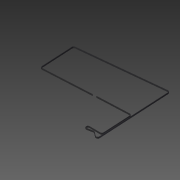
# Autodesk Inventor part: BeltLeft
Saved by Autodesk Inventor 2015 (Build 190159000, 159)
## iProperties
Company: RobotDigg
Created: 2014-08-13
Part Number: BeltLeft
Material: Rubber, Silicone
Document SubType Name: Modeling
Designer: Jack
Density: 1.25 g/cm^3
Appearance: Rubber - Black - Version 1.1
Author: Jack
Autodesk Inventor part; units mm, degrees
ref_plane "YZ Plane" through (0, 0, 0) normal (1, 0, 0) x (0, 1, 0)
ref_plane "XZ Plane" through (0, 0, 0) normal (0, 1, 0) x (-1, 0, 0)
ref_plane "XY Plane" through (0, 0, 0) normal (0, 0, 1) x (1, 0, 0)
sketch "Sketch1" plane through (0, 0, 0) normal (0, 0, 1) x (1, 0, 0)
  circle A0 centre (0, 0) radius 7.5 projected
  circle A1 centre (54.6789, -11.0553) radius 6.5 projected
  circle A2 centre (48.3325, 13.6372) radius 6.5 projected
  circle A3 centre (41.6146, 137.5136) radius 6.5 projected
  circle A4 centre (37.1883, 311.4708) radius 6.5 projected
  circle A5 centre (-336.2868, 273.1908) radius 6.5 projected
  circle A6 centre (-328.6547, 132.4559) radius 6.5 projected
  circle A7 centre (28.0291, -9.0111) radius 6.5 projected
  line L0 (0.0451, 5.9998) -> (48.2723, 5.6375)
  arc A8 (48.2723, 5.6375) -> (56.3207, 14.0704) centre (48.3325, 13.6372) ccw
  line L1 (56.3207, 14.0704) -> (49.6029, 137.9468)
  arc A9 (49.6029, 137.9468) -> (41.2546, 145.5055) centre (41.6146, 137.5136) ccw
  line L2 (61.1693, -10.7034) -> (43.6788, 311.8227)
  line L3 (36.5255, 317.9369) -> (-336.9495, 279.6569)
  line L4 (-342.7773, 272.8388) -> (-335.1452, 132.1039)
  line L5 (-328.3027, 125.9655) -> (-115.5574, 137.504)
  line L6 (50.7453, -16.23) -> (32.8704, -2.6423)
  arc A10 (32.8704, -2.6423) -> (26.5615, -1.1469) centre (28.0291, -9.0111) ccw
  line L7 (26.5615, -1.1469) -> (1.1007, -5.8982)
  arc A11 (0.0451, 5.9998) -> (1.1007, -5.8982) centre (0, 0) ccw
  arc A12 (50.7453, -16.23) -> (61.1693, -10.7034) centre (54.6789, -11.0553) ccw
  arc A13 (43.6788, 311.8227) -> (36.5255, 317.9369) centre (37.1883, 311.4708) ccw
  arc A14 (-336.9495, 279.6569) -> (-342.7773, 272.8388) centre (-336.2868, 273.1908) ccw
  arc A15 (-335.1452, 132.1039) -> (-328.3027, 125.9655) centre (-328.6547, 132.4559) ccw
  line L8 (41.2546, 145.5055) -> (-99.9128, 139.1455)
  line L9 (-99.9128, 137.6439) -> (41.3221, 144.007)
  arc A16 (48.1051, 137.8655) -> (41.3221, 144.007) centre (41.6146, 137.5136) ccw
  line L10 (48.1051, 137.8655) -> (54.8229, 13.9892)
  arc A17 (48.2836, 7.1374) -> (54.8229, 13.9892) centre (48.3325, 13.6372) ccw
  line L11 (48.2836, 7.1374) -> (0.0564, 7.4998)
  arc A18 (0.0564, 7.4998) -> (1.3758, -7.3727) centre (0, 0) ccw
  line L12 (1.3758, -7.3727) -> (26.8367, -2.6214)
  arc A19 (31.9626, -3.8365) -> (26.8367, -2.6214) centre (28.0291, -9.0111) ccw
  line L13 (31.9626, -3.8365) -> (49.8376, -17.4242)
  arc A20 (49.8376, -17.4242) -> (62.6671, -10.6221) centre (54.6789, -11.0553) ccw
  line L14 (62.6671, -10.6221) -> (45.1766, 311.904)
  arc A21 (45.1766, 311.904) -> (36.3726, 319.4291) centre (37.1883, 311.4708) ccw
  line L15 (36.3726, 319.4291) -> (-337.1025, 281.1491)
  arc A22 (-337.1025, 281.1491) -> (-344.2751, 272.7576) centre (-336.2868, 273.1908) ccw
  line L16 (-344.2751, 272.7576) -> (-336.643, 132.0227)
  arc A23 (-336.643, 132.0227) -> (-328.2215, 124.4677) centre (-328.6547, 132.4559) ccw
  line L17 (-328.2215, 124.4677) -> (-115.5574, 136.0018)
  line L18 (-99.9128, 137.6439) -> (-99.9128, 139.1455)
  line L19 (-115.5574, 136.0018) -> (-115.5574, 137.504)
  dimension "d0" = 1.5
  dimension "d1" = 1.5
  dimension "d2" = 1.5
  dimension "d3" = 1.5
  dimension "d6" = 6
  constraints: 40 end point, 40 point on circle, 20 tangent, 16 centre point, 4 coincident, 3 concentric, 1 parallel, 1 vertical, 16 other
  measures "d0" radial gap between concentric circles of A8 A2
  measures "d1" radial gap between concentric circles of A3 A9
  measures "d2" radial gap between concentric circles of A7 A10
  measures "d3" distance between parallel lines of L0 L11
  measures "d6" radius of A11
extrude "Extrusion1" add sketch "Sketch1" along normal blind 6 contours A0 L0 A11 L7 | L11 A2 L10 A3 L9 L18 L8 A9 L1 A8 L0 A0 | A0 L7 A10 L6 A1 L2 A4 L3 A5 L4 A6 L5 L19 L17 A23 L16 A22 L15 A21 L14 A20 L13 A7 L12 picked at (2.587, 6.2542)
body "Solid1"
